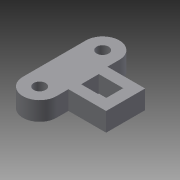
# Autodesk Inventor part: LinesensorHolderTopRound
Saved by Autodesk Inventor 2015 (Build 190159000, 159)
## iProperties
Created: 2017-02-01
Part Number: LinesensorHolderTopRound
Material: Generic
Document SubType Name: Modeling
Designer: Ernest
Density: 1 g/cm^3
Appearance: Default
Author: Ernest
Autodesk Inventor part; units mm, degrees
ref_plane "YZ Plane" through (0, 0, 0) normal (1, 0, 0) x (0, 1, 0)
ref_plane "XZ Plane" through (0, 0, 0) normal (0, 1, 0) x (-1, 0, 0)
ref_plane "XY Plane" through (0, 0, 0) normal (0, 0, 1) x (1, 0, 0)
sketch "Sketch1" plane through (0, 0, 0) normal (0, 1, 0) x (-1, 0, 0)
  line L0 (0, 0) -> (4.6, 0)
  line L1 (4.6, 0) -> (4.6, 10.16)
  line L2 (4.6, 10.16) -> (6, 10.16)
  line L3 (6, 10.16) -> (6, 0)
  line L4 (6, 0) -> (10.6, 0)
  line L5 (10.6, 0) -> (10.6, 14)
  line L6 (10.6, 14) -> (0, 14)
  line L7 (0, 14) -> (0, 0)
  dimension "d0" = 1.4
  dimension "d1" = 10.16
  dimension "d2" = 14
  dimension "d3" = 4.6
  constraints: 16 end point, 6 perpendicular, 2 point on line, 1 collinear, 1 horizontal
  measures "d0" distance between parallel lines of L1 L3
  measures "d1" distance of L2.end L3.end
  measures "d2" distance of L4.end L5.end
  measures "d3" distance of L0.start L0.end
extrude "Extrusion1" add sketch "Sketch1" along normal blind 10.4
sketch "Sketch2" plane through (0, 0, 14) normal (1, 0, 0) x (0, 0, -1)
  line L0 (0, 0) -> (14, 0) projected
  line L1 (14, 0) -> (14, 10.4) projected
  line L2 (0, 10.4) -> (14, 10.4) projected
  line L3 (0, 0) -> (0, 10.4) projected
  line L4 (4.5, 7.55) -> (11, 7.55)
  line L5 (11, 7.55) -> (11, 2.85)
  line L6 (11, 2.85) -> (4.5, 2.85)
  line L7 (4.5, 2.85) -> (4.5, 7.55)
  dimension "d6" = 3
  dimension "d7" = 6.5
  dimension "d8" = 4.7
  dimension "d9" = 2.85
  dimension "d12" = 10.4
  constraints: 8 end point, 2 parallel, 1 horizontal, 1 perpendicular
  measures "d6" distance between parallel lines of L1 L5
  measures "d7" distance of L4.start L4.end
  measures "d8" distance of L6.end L4.start
  measures "d9" distance between parallel lines of L2 L4
  measures "d12" distance of L0.end L1.end
extrude "Extrusion2" cut sketch "Sketch2" against normal blind 12.4 contours L4 L5 L6 L7
sketch "Sketch3" plane through (-6, 0, 10.16) normal (1, 0, 0) x (0, 0, -1)
  line L0 (0.66, 2.85) -> (0.66, 7.55) projected
  line L1 (0.66, 7.55) -> (7.16, 7.55) projected
  line L2 (7.16, 7.55) -> (7.16, 2.85) projected
  line L3 (7.16, 2.85) -> (0.66, 2.85) projected
  line L4 (0, 0) -> (10.16, 0) projected
  line L5 (10.16, 0) -> (10.16, 10.4) projected
  line L6 (0, 10.4) -> (10.16, 10.4) projected
  line L7 (0, 0) -> (0, 10.4) projected
  line L8 (0.81, 7.4) -> (7.01, 7.4)
  line L9 (7.01, 7.4) -> (7.01, 3)
  line L10 (7.01, 3) -> (0.81, 3)
  line L11 (0.81, 3) -> (0.81, 7.4)
  dimension "d13" = 0.15
  dimension "d14" = 0.15
  dimension "d16" = 0.15
  dimension "d17" = 0.15
  constraints: 8 end point, 2 parallel, 1 horizontal, 1 perpendicular
  measures "d13" distance between parallel lines of L3 L10
  measures "d14" distance between parallel lines of L2 L9
  measures "d16" distance between parallel lines of L1 L8
  measures "d17" distance between parallel lines of L0 L11
extrude "Extrusion3" add sketch "Sketch3" against normal blind 0.1 contours L0 L1 L2 L3
fillet "Fillet1" radius 0.15 4 edges at (-6.1, 5.2, 3) (-6.1, 5.2, 9.5) (-6.1, 2.85, 6.25) (-6.1, 7.55, 6.25)
sketch "Sketch4" plane through (-4.6, 0, 0) normal (-1, 0, 0) x (0, 0, 1)
  line L0 (9.5, 7.55) -> (9.5, 2.85) projected
  line L1 (9.5, 2.85) -> (3, 2.85) projected
  line L2 (3, 2.85) -> (3, 7.55) projected
  line L3 (3, 7.55) -> (9.5, 7.55) projected
  line L4 (0, 0) -> (10.16, 0) projected
  line L5 (10.16, 0) -> (10.16, 10.4) projected
  line L6 (0, 10.4) -> (10.16, 10.4) projected
  line L7 (0, 0) -> (0, 10.4) projected
  line L8 (3.15, 7.4) -> (9.35, 7.4)
  line L9 (9.35, 7.4) -> (9.35, 3)
  line L10 (9.35, 3) -> (3.15, 3)
  line L11 (3.15, 3) -> (3.15, 7.4)
  dimension "d21" = 0.15
  dimension "d22" = 0.15
  dimension "d23" = 0.15
  dimension "d24" = 0.15
  constraints: 8 end point, 2 parallel, 1 horizontal, 1 perpendicular
  measures "d21" distance between parallel lines of L2 L11
  measures "d22" distance between parallel lines of L3 L8
  measures "d23" distance between parallel lines of L1 L10
  measures "d24" distance between parallel lines of L0 L9
extrude "Extrusion4" add sketch "Sketch4" against normal blind 0.1 contours L0 L1 L2 L3
fillet "Fillet2" radius 0.15 4 edges at (-4.5, 5.2, 9.5) (-4.5, 2.85, 6.25) (-4.5, 7.55, 6.25) (-4.5, 5.2, 3)
sketch "Sketch5" plane through (-10.6, 0, 14) normal (0, 0, 1) x (1, 0, 0)
  line L0 (0, 0) -> (10.6, 0) projected
  line L1 (10.6, 0) -> (10.6, 10.4) projected
  line L2 (0, 10.4) -> (10.6, 10.4) projected
  line L3 (0, 0) -> (0, 10.4) projected
  point P0 (10.6, 0)
extrude "Extrusion5" add sketch "Sketch5" along normal blind 5
sketch "Sketch18" plane through (-6, 0, 10.16) normal (1, 0, 0) x (0, 0, -1)
  line L0 (0.81, 3) -> (0.81, 7.4) projected
  line L1 (0.81, 7.4) -> (7.01, 7.4) projected
  line L2 (7.01, 7.4) -> (7.01, 3) projected
  line L3 (7.01, 3) -> (0.81, 3) projected
  line L4 (0, 0) -> (10.16, 0) projected
  line L5 (10.16, 0) -> (10.16, 10.4) projected
  line L6 (0, 10.4) -> (10.16, 10.4) projected
  line L7 (0, 0) -> (0, 10.4) projected
  line L8 (0.66, 7.55) -> (7.16, 7.55) projected
  line L9 (7.16, 7.55) -> (0.66, 7.55) projected
  line L10 (7.16, 7.55) -> (7.16, 2.85) projected
  line L11 (7.16, 2.85) -> (7.16, 7.55) projected
  line L12 (0.66, 2.85) -> (0.66, 7.55) projected
  line L13 (0.66, 7.55) -> (0.66, 2.85) projected
  line L14 (7.16, 2.85) -> (0.66, 2.85) projected
  line L15 (0.66, 2.85) -> (7.16, 2.85) projected
  line L16 (7.16, 7.55) -> (0.66, 7.55)
  line L17 (0.66, 7.55) -> (0.66, 2.85)
  line L18 (0.66, 2.85) -> (7.16, 2.85)
  line L19 (7.16, 2.85) -> (7.16, 7.55)
  line L20 (5.76, 6.95) -> (2.06, 6.95)
  line L21 (2.06, 6.95) -> (2.06, 5.45)
  line L22 (2.06, 5.45) -> (5.76, 5.45)
  line L23 (5.76, 5.45) -> (5.76, 6.95)
  line L24 (5.76, 4.95) -> (2.06, 4.95)
  line L25 (2.06, 4.95) -> (2.06, 3.45)
  line L26 (2.06, 3.45) -> (5.76, 3.45)
  line L27 (5.76, 3.45) -> (5.76, 4.95)
  line L28 (7.16, 2.85) -> (7.16, 7.55) projected
  line L29 (0.66, 2.85) -> (0.66, 7.55) projected
  line L30 (0.66, 5.2) -> (20.66, 5.2) construction
  line L31 (20.66, 5.2) -> (5.76, 4.6797)
  line L32 (20.66, 5.2) -> (5.76, 5.7203)
  line L33 (20.66, 5.2) -> (5.76, 3.7981)
  line L34 (20.66, 5.2) -> (5.76, 6.6019)
  line L35 (5.76, 3.7981) -> (2.06, 3.45)
  line L36 (2.06, 3.45) -> (0.81, 3.3324)
  line L37 (5.76, 4.6797) -> (2.06, 4.5505)
  line L38 (2.06, 4.5505) -> (0.81, 4.5068)
  line L39 (2.06, 5.8495) -> (0.81, 5.8932)
  line L40 (5.76, 5.7203) -> (2.06, 5.8495)
  line L41 (2.06, 6.95) -> (0.81, 7.0676)
  line L42 (5.76, 6.6019) -> (2.06, 6.95)
  dimension "d79" = 3.7
  dimension "d80" = 6.5
  dimension "d81" = 1.4
  dimension "d82" = 1.5
  dimension "d83" = 2
  dimension "d85" = 20
  dimension "d86" = 4
  dimension "d87" = 2
  dimension "d88" = 0.25
  constraints: 50 end point, 13 point on line, 6 parallel, 4 horizontal, 3 perpendicular, 1 collinear, 2 other
  measures "d79" distance of L20.start L20.end
  measures "d80" distance of L9.start L9.end
  measures "d81" distance between parallel lines of L23 L10
  measures "d82" distance of L22.end L20.start
  measures "d83" distance between parallel lines of L24 L20
  measures "d85" distance of L30.start L30.end
  measures "d86" angle of L32 L31
  measures "d87" angle of L30 L31
  measures "d88" distance between parallel lines of L30 L22
extrude "Extrusion18" add sketch "Sketch18" against normal blind 0.4 contours L0 L36 L26 L27 L33 L2 L3 | L0 L38 L25 L36 | L0 L39 L21 L22 L23 L32 L2 L31 L27 L24 L25 L38 | L35 L27 L26 | L33 L27 L31 L2 | L0 L41 L21 L39 | L25 L24 L27 L37 | L0 L1 L2 L34 L23 L20 L41 | L40 L23 L22 L21 | L32 L23 L34 L2 | L20 L23 L42
sketch "Sketch19" plane through (-10.6, 0, 0) normal (-1, 0, 0) x (0, 0, 1)
  line L0 (9.5, 7.55) -> (9.5, 2.85) projected
  line L1 (9.5, 2.85) -> (3, 2.85) projected
  line L2 (3, 2.85) -> (3, 7.55) projected
  line L3 (3, 7.55) -> (9.5, 7.55) projected
  line L4 (0, 0) -> (19, 0) projected
  line L5 (19, 10.4) -> (19, 0) projected
  line L6 (0, 10.4) -> (19, 10.4) projected
  line L7 (0, 0) -> (0, 10.4) projected
  point P0 (0, 0)
extrude "Extrusion19" add sketch "Sketch19" along normal blind 0.4
sketch "Sketch20" plane through (-11, 0, 0) normal (-1, 0, 0) x (0, 0, 1)
  line L0 (9.5, 2.85) -> (3, 2.85) projected
  line L1 (3, 2.85) -> (3, 7.55) projected
  line L2 (3, 7.55) -> (9.5, 7.55) projected
  line L3 (9.5, 7.55) -> (9.5, 2.85) projected
  line L4 (0, 0) -> (19, 0) projected
  line L5 (19, 0) -> (19, 10.4) projected
  line L6 (19, 10.4) -> (0, 10.4) projected
  line L7 (0, 10.4) -> (0, 0) projected
  circle A0 centre (14.5251, -3.2) radius 1.6
  circle A1 centre (14.5251, 13.6) radius 1.6
  arc A2 (10.0502, -3.2) -> (19, -3.2) centre (14.5251, -3.2) ccw
  arc A3 (19, 13.6) -> (10.0502, 13.6) centre (14.5251, 13.6) ccw
  line L8 (19, -3.2) -> (19, 13.6)
  line L9 (10.0502, -3.2) -> (10.0502, 13.6)
  point P0 (0, 0)
  dimension "d97" = 3.2
  dimension "d98" = 3.2
  dimension "d99" = 3.2
  dimension "d100" = 3.2
  constraints: 4 centre point, 4 end point, 4 point on circle, 3 tangent, 2 coincident, 1 vertical
  measures "d97" diameter of A0
  measures "d98" diameter of A1
  measures "d99" distance from line of L4 A0.centre
  measures "d100" distance from line of L6 A1.centre
extrude "Extrusion20" add sketch "Sketch20" against normal blind 11 contours L9 L6 L5 L4 | L4 L8 A2 L9 | L9 A3 L8 L6
sketch "Sketch21" plane through (-6, 0, 0) normal (0, 0, -1) x (-1, 0, 0)
  line L0 (0, 10.4) -> (0, 0) projected
  line L1 (0, 0) -> (0, 10.4) projected
  line L2 (0, 3.45) -> (0, 4.5505) projected
  line L3 (0, 4.5505) -> (0, 4.6797) projected
  line L4 (0, 4.6797) -> (0, 3.7981) projected
  line L5 (0, 3.7981) -> (0, 3.45) projected
  line L6 (0, 5.8495) -> (0, 6.95) projected
  line L7 (0, 6.95) -> (0, 6.6019) projected
  line L8 (0, 6.6019) -> (0, 5.7203) projected
  line L9 (0, 5.7203) -> (0, 5.8495) projected
  line L10 (-1.4, 0) -> (-1.4, 10.4) projected
  line L11 (-1.4, 0) -> (-1.4, 10.4) projected
  line L12 (-1.4, 3) -> (-1.4, 7.4) projected
  line L13 (-1.4, 7.4) -> (-1.4, 3) projected
  line L14 (0, 19.9203) -> (-9.948, 19.9203)
  line L15 (-9.948, 19.9203) -> (-9.948, -11.4831)
  line L16 (-9.948, -11.4831) -> (0, -11.4831)
  line L17 (0, -11.4831) -> (0, 19.9203)
  point P0 (-6, 0)
  constraints: 8 end point, 2 parallel, 1 horizontal, 1 perpendicular
extrude "Extrusion21" cut sketch "Sketch21" against normal blind 32.75
sketch "Sketch22" plane through (-6.4, 0, 10.16) normal (-1, 0, 0) x (0, 0, 1)
  line L0 (-0.81, 3) -> (-0.81, 7.4) projected
  line L1 (-0.81, 7.4) -> (-7.01, 7.4) projected
  line L2 (-7.01, 7.4) -> (-7.01, 3) projected
  line L3 (-7.01, 3) -> (-0.81, 3) projected
  line L4 (-2.06, 6.95) -> (-2.06, 5.8495) projected
  line L5 (-2.06, 5.8495) -> (-5.76, 5.7203) projected
  line L6 (-5.76, 5.7203) -> (-5.76, 6.6019) projected
  line L7 (-5.76, 6.6019) -> (-2.06, 6.95) projected
  line L8 (-2.06, 4.5505) -> (-2.06, 3.45) projected
  line L9 (-2.06, 3.45) -> (-5.76, 3.7981) projected
  line L10 (-5.76, 3.7981) -> (-5.76, 4.6797) projected
  line L11 (-5.76, 4.6797) -> (-2.06, 4.5505) projected
  line L12 (-0.4526, 7.7559) -> (-7.5346, 7.7559)
  line L13 (-7.5346, 7.7559) -> (-7.5346, 2.5335)
  line L14 (-7.5346, 2.5335) -> (-0.4526, 2.5335)
  line L15 (-0.4526, 2.5335) -> (-0.4526, 7.7559)
  point P0 (-10.16, 0)
  constraints: 8 end point, 2 parallel, 1 horizontal, 1 perpendicular
extrude "Extrusion22" add sketch "Sketch22" against normal up to surface (0.4 mm away) contours L3 L2 L1 L0 | L15 L14 L13 L12
extrude "Extrusion23" add sketch "Sketch22" along normal blind 0.1 contours L3 L2 L1 L0 | L15 L14 L13 L12
equation "\"d9\" = -0.5 * d8 + 0.5 * d12"
equation "\"d81\" = -0.5 * d79 + 0.5 * d80"
equation "\"d87\" = 0.5 * d86"
body "Solid1"
